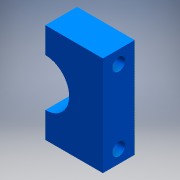
# Autodesk Inventor part: Semi Cuscinetto
Saved by Autodesk Inventor 2016 (Build 200138000, 138)
## iProperties
Created: 2016-09-09
Part Number: Semi Cuscinetto
Material: Generic
Document SubType Name: Modeling
Designer: Muhammad
Density: 1 g/cm^3
Appearance: Default
Author: Muhammad
Autodesk Inventor part; units mm, degrees
ref_plane "YZ Plane" through (0, 0, 0) normal (1, 0, 0) x (0, 1, 0)
ref_plane "XZ Plane" through (0, 0, 0) normal (0, 1, 0) x (-1, 0, 0)
ref_plane "XY Plane" through (0, 0, 0) normal (0, 0, 1) x (1, 0, 0)
sketch "Sketch1" plane through (0, 0, 0) normal (0, 1, 0) x (-1, 0, 0)
  arc A0 (0, 6) -> (0, -6) centre (0, 0) ccw
  line L0 (0, 0) -> (-14.5, 0) construction
  line L1 (0, 6) -> (0, 12.5)
  line L2 (0, 12.5) -> (-14.5, 12.5)
  line L3 (0, -6) -> (0, -12.5)
  line L4 (0, -12.5) -> (-14.5, -12.5)
  line L5 (-14.5, 12.5) -> (-14.5, -12.5)
  constraints: 12 end point, 3 vertical, 2 perpendicular, 2 point on circle, 1 centre point, 1 coincident, 1 horizontal
extrude "Extrusion1" add sketch "Sketch1" along normal blind 8
sketch "Sketch2" plane through (0, 8, 0) normal (0, 1, 0) x (1, 0, 0)
  line L0 (14.5, -12.5) -> (14.5, 12.5) construction
  line L1 (0, 12.5) -> (0, 6) construction
  line L2 (0, -6) -> (0, -12.5) construction
  point P0 (0, 0)
sketch "Sketch3" plane through (0, 0, -12.5) normal (-1, 0, 0) x (0, 0, 1)
  line L0 (0, 8) -> (6.5, 8) construction
  line L1 (3.25, 8) -> (3.25, 0) construction
  line L2 (25, 8) -> (0, 8) construction
  line L3 (18.5, 8) -> (25, 8) construction
  line L4 (21.75, 8) -> (21.75, 0) construction
  line L5 (12.5, 0) -> (12.5, 8) construction
  line L6 (25, 0) -> (25, 8) construction
  line L7 (25, 4) -> (0, 4) construction
  line L8 (0, 0) -> (0, 8) construction
  circle A0 centre (21.75, 4) radius 1.6
  circle A1 centre (3.25, 4) radius 1.6
  dimension "d8" = 3.2
  dimension "d9" = 3.2
  constraints: 8 end point, 7 midpoint, 2 centre point, 2 point on line, 1 perpendicular, 1 vertical
  measures "d8" diameter of A0
  measures "d9" diameter of A1
extrude "Extrusion2" cut sketch "Sketch3" against normal through all
sketch "Sketch4" plane through (0, 8, 0) normal (0, 1, 0) x (1, 0, 0)
  point P0 (0, 0)
body "Solid1"
